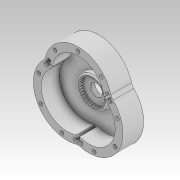
# Autodesk Inventor part: Housing
Saved by Autodesk Inventor 2020 (Build 240168000, 168)
## iProperties
Created: 2022-01-08
Part Number: Housing
Material: Generic
Document SubType Name: Modeling
Designer: DDeGo
Density: 1 g/cm^3
Appearance: Default
Author: DDeGo
Autodesk Inventor part; units mm, degrees
(part 1 of 2)
ref_plane "YZ Plane" through (0, 0, 0) normal (1, 0, 0) x (0, 1, 0)
ref_plane "XZ Plane" through (0, 0, 0) normal (0, 1, 0) x (-1, 0, 0)
ref_plane "XY Plane" through (0, 0, 0) normal (0, 0, 1) x (1, 0, 0)
sketch "Block1" plane through (0, 0, 0) normal (0, 0, 1) x (1, 0, 0)
  arc A0 (4.8525, -6.0461) -> (5.1116, -5.8287) centre (0, 0) ccw
  arc A1 (4.1606, -5.6743) -> (4.8525, -6.0461) centre (5.9978, -3.0847) ccw
  arc A2 (3.9091, -5.8504) -> (4.1606, -5.6743) centre (0, 0) ccw
  arc A3 (4.0218, -6.6277) -> (3.9091, -5.8504) centre (0.8473, -6.6911) ccw
  arc A4 (3.7289, -6.7968) -> (4.0218, -6.6277) centre (0, 0) ccw
  arc A5 (3.112, -6.3106) -> (3.7289, -6.7968) centre (5.371, -4.0793) ccw
  arc A6 (2.8338, -6.4403) -> (3.112, -6.3106) centre (0, 0) ccw
  arc A7 (2.8098, -7.2254) -> (2.8338, -6.4403) centre (-0.3275, -6.7366) ccw
  arc A8 (2.492, -7.3411) -> (2.8098, -7.2254) centre (0, 0) ccw
  arc A9 (2.8367, -7.2471) -> (2.8656, -6.4591) centre (-0.3275, -6.7366) ccw
  arc A10 (2.8656, -6.4591) -> (3.1059, -6.347) centre (0, 0) ccw
  arc A11 (3.1059, -6.347) -> (3.7282, -6.8314) centre (5.371, -4.0793) ccw
  arc A12 (3.7282, -6.8314) -> (4.0521, -6.6444) centre (0, 0) ccw
  arc A13 (4.0521, -6.6444) -> (3.9437, -5.8633) centre (0.8473, -6.6911) ccw
  arc A14 (3.9437, -5.8633) -> (4.1609, -5.7112) centre (0, 0) ccw
  arc A15 (4.1609, -5.7112) -> (4.8578, -6.0802) centre (5.9978, -3.0847) ccw
  arc A16 (4.8578, -6.0802) -> (5.1443, -5.8398) centre (0, 0) ccw
  arc A17 (2.4853, -7.375) -> (2.8367, -7.2471) centre (0, 0) ccw
  arc A18 (6.0461, -4.8525) -> (5.6743, -4.1606) centre (3.0847, -5.9978) ccw
  arc A19 (6.0802, -4.8578) -> (5.7112, -4.1609) centre (3.0847, -5.9978) ccw
  arc A20 (5.8287, -5.1116) -> (6.0461, -4.8525) centre (0, 0) ccw
  arc A21 (5.8398, -5.1443) -> (6.0802, -4.8578) centre (0, 0) ccw
  arc A22 (5.0827, -4.8656) -> (5.8287, -5.1116) centre (6.4423, -1.9963) ccw
  arc A23 (5.0894, -4.9019) -> (5.8398, -5.1443) centre (6.4423, -1.9963) ccw
  arc A24 (4.9019, -5.0894) -> (5.0894, -4.9019) centre (0, 0) ccw
  arc A25 (4.8656, -5.0827) -> (5.0827, -4.8656) centre (0, 0) ccw
  arc A26 (5.1443, -5.8398) -> (4.9019, -5.0894) centre (1.9963, -6.4423) ccw
  arc A27 (5.1116, -5.8287) -> (4.8656, -5.0827) centre (1.9963, -6.4423) ccw
  arc A28 (1.9689, -6.7551) -> (2.492, -7.3411) centre (4.5811, -4.95) ccw
  arc A29 (1.6724, -6.8346) -> (1.9689, -6.7551) centre (0, 0) ccw
  arc A30 (1.5124, -7.6036) -> (1.6724, -6.8346) centre (-1.4923, -6.5774) ccw
  arc A31 (1.1793, -7.6623) -> (1.5124, -7.6036) centre (0, 0) ccw
  arc A32 (0.7478, -7.0265) -> (1.1669, -7.6945) centre (3.6519, -5.6703) ccw
  arc A33 (0.766, -6.9944) -> (1.1793, -7.6623) centre (3.6519, -5.6703) ccw
  arc A34 (1.1669, -7.6945) -> (1.5352, -7.6296) centre (0, 0) ccw
  arc A35 (1.5352, -7.6296) -> (1.7005, -6.8585) centre (-1.4923, -6.5774) ccw
  arc A36 (1.7005, -6.8585) -> (1.9566, -6.7899) centre (0, 0) ccw
  arc A37 (1.9566, -6.7899) -> (2.4853, -7.375) centre (4.5811, -4.95) ccw
  arc A38 (5.7112, -4.1609) -> (5.8633, -3.9437) centre (0, 0) ccw
  arc A39 (5.6743, -4.1606) -> (5.8504, -3.9091) centre (0, 0) ccw
  arc A40 (5.8633, -3.9437) -> (6.6444, -4.0521) centre (6.6911, -0.8473) ccw
  arc A41 (5.8504, -3.9091) -> (6.6277, -4.0218) centre (6.6911, -0.8473) ccw
  arc A42 (6.6444, -4.0521) -> (6.8314, -3.7282) centre (0, 0) ccw
  arc A43 (6.7968, -3.7289) -> (6.3106, -3.112) centre (4.0793, -5.371) ccw
  arc A44 (6.8314, -3.7282) -> (6.347, -3.1059) centre (4.0793, -5.371) ccw
  arc A45 (6.6277, -4.0218) -> (6.7968, -3.7289) centre (0, 0) ccw
  arc A46 (-0.1691, -7.7507) -> (0.1691, -7.7507) centre (0, 0) ccw
  arc A47 (-0.4602, -7.0211) -> (-0.1691, -7.7507) centre (2.6118, -6.2183) ccw
  arc A48 (-1.7005, -6.8585) -> (-1.5352, -7.6296) centre (1.4923, -6.5774) ccw
  arc A49 (-1.6724, -6.8346) -> (-1.5124, -7.6036) centre (1.4923, -6.5774) ccw
  arc A50 (-1.5124, -7.6036) -> (-1.1793, -7.6623) centre (0, 0) ccw
  arc A51 (-1.1793, -7.6623) -> (-0.766, -6.9944) centre (-3.6519, -5.6703) ccw
  arc A52 (-1.1669, -7.6945) -> (-0.7478, -7.0265) centre (-3.6519, -5.6703) ccw
  arc A53 (-0.7478, -7.0265) -> (-0.4837, -7.0496) centre (0, 0) ccw
  arc A54 (-0.766, -6.9944) -> (-0.4602, -7.0211) centre (0, 0) ccw
  arc A55 (-0.4837, -7.0496) -> (-0.187, -7.7803) centre (2.6118, -6.2183) ccw
  arc A56 (0.4602, -7.0211) -> (0.766, -6.9944) centre (0, 0) ccw
  arc A57 (0.4837, -7.0496) -> (0.7478, -7.0265) centre (0, 0) ccw
  arc A58 (0.1691, -7.7507) -> (0.4602, -7.0211) centre (-2.6118, -6.2183) ccw
  arc A59 (0.187, -7.7803) -> (0.4837, -7.0496) centre (-2.6118, -6.2183) ccw
  arc A60 (-0.187, -7.7803) -> (0.187, -7.7803) centre (0, 0) ccw
  arc A61 (-1.5352, -7.6296) -> (-1.1669, -7.6945) centre (0, 0) ccw
  arc A62 (-1.9566, -6.7899) -> (-1.7005, -6.8585) centre (0, 0) ccw
  arc A63 (-1.9689, -6.7551) -> (-1.6724, -6.8346) centre (0, 0) ccw
  arc A64 (-2.4853, -7.375) -> (-1.9566, -6.7899) centre (-4.5811, -4.95) ccw
  arc A65 (-2.492, -7.3411) -> (-1.9689, -6.7551) centre (-4.5811, -4.95) ccw
  arc A66 (6.9944, -0.766) -> (7.0211, -0.4602) centre (0, 0) ccw
  arc A67 (7.6623, -1.1793) -> (6.9944, -0.766) centre (5.6703, -3.6519) ccw
  arc A68 (7.6036, -1.5124) -> (7.6623, -1.1793) centre (0, 0) ccw
  arc A69 (6.8346, -1.6724) -> (7.6036, -1.5124) centre (6.5774, 1.4923) ccw
  arc A70 (6.7551, -1.9689) -> (6.8346, -1.6724) centre (0, 0) ccw
  arc A71 (7.3411, -2.492) -> (6.7551, -1.9689) centre (4.95, -4.5811) ccw
  arc A72 (7.2254, -2.8098) -> (7.3411, -2.492) centre (0, 0) ccw
  arc A73 (6.4403, -2.8338) -> (7.2254, -2.8098) centre (6.7366, 0.3275) ccw
  arc A74 (6.3106, -3.112) -> (6.4403, -2.8338) centre (0, 0) ccw
  arc A75 (6.4591, -2.8656) -> (7.2471, -2.8367) centre (6.7366, 0.3275) ccw
  arc A76 (7.2471, -2.8367) -> (7.375, -2.4853) centre (0, 0) ccw
  arc A77 (6.7899, -1.9566) -> (6.8585, -1.7005) centre (0, 0) ccw
  arc A78 (7.375, -2.4853) -> (6.7899, -1.9566) centre (4.95, -4.5811) ccw
  arc A79 (6.8585, -1.7005) -> (7.6296, -1.5352) centre (6.5774, 1.4923) ccw
  arc A80 (7.6296, -1.5352) -> (7.6945, -1.1669) centre (0, 0) ccw
  arc A81 (7.6945, -1.1669) -> (7.0265, -0.7478) centre (5.6703, -3.6519) ccw
  arc A82 (7.0265, -0.7478) -> (7.0496, -0.4837) centre (0, 0) ccw
  arc A83 (6.347, -3.1059) -> (6.4591, -2.8656) centre (0, 0) ccw
  arc A84 (-3.9091, -5.8504) -> (-4.0218, -6.6277) centre (-0.8473, -6.6911) ccw
  arc A85 (-4.0218, -6.6277) -> (-3.7289, -6.7968) centre (0, 0) ccw
  arc A86 (-4.0521, -6.6444) -> (-3.7282, -6.8314) centre (0, 0) ccw
  arc A87 (-3.1059, -6.347) -> (-2.8656, -6.4591) centre (0, 0) ccw
  arc A88 (-3.7289, -6.7968) -> (-3.112, -6.3106) centre (-5.371, -4.0793) ccw
  arc A89 (-3.112, -6.3106) -> (-2.8338, -6.4403) centre (0, 0) ccw
  arc A90 (-3.7282, -6.8314) -> (-3.1059, -6.347) centre (-5.371, -4.0793) ccw
  arc A91 (-2.8338, -6.4403) -> (-2.8098, -7.2254) centre (0.3275, -6.7366) ccw
  arc A92 (-2.8656, -6.4591) -> (-2.8367, -7.2471) centre (0.3275, -6.7366) ccw
  arc A93 (-2.8098, -7.2254) -> (-2.492, -7.3411) centre (0, 0) ccw
  arc A94 (-2.8367, -7.2471) -> (-2.4853, -7.375) centre (0, 0) ccw
  arc A95 (-3.9437, -5.8633) -> (-4.0521, -6.6444) centre (-0.8473, -6.6911) ccw
  arc A96 (-4.1609, -5.7112) -> (-3.9437, -5.8633) centre (0, 0) ccw
  arc A97 (-4.8578, -6.0802) -> (-4.1609, -5.7112) centre (-5.9978, -3.0847) ccw
  arc A98 (-4.8525, -6.0461) -> (-4.1606, -5.6743) centre (-5.9978, -3.0847) ccw
  arc A99 (-5.1116, -5.8287) -> (-4.8525, -6.0461) centre (0, 0) ccw
  arc A100 (-5.1443, -5.8398) -> (-4.8578, -6.0802) centre (0, 0) ccw
  arc A101 (-4.8656, -5.0827) -> (-5.1116, -5.8287) centre (-1.9963, -6.4423) ccw
  arc A102 (-4.9019, -5.0894) -> (-5.1443, -5.8398) centre (-1.9963, -6.4423) ccw
  arc A103 (-4.1606, -5.6743) -> (-3.9091, -5.8504) centre (0, 0) ccw
  arc A104 (6.8346, 1.6724) -> (6.7551, 1.9689) centre (0, 0) ccw
  arc A105 (7.6036, 1.5124) -> (6.8346, 1.6724) centre (6.5774, -1.4923) ccw
  arc A106 (7.6623, 1.1793) -> (7.6036, 1.5124) centre (0, 0) ccw
  arc A107 (6.9944, 0.766) -> (7.6623, 1.1793) centre (5.6703, 3.6519) ccw
  arc A108 (7.0211, 0.4602) -> (6.9944, 0.766) centre (0, 0) ccw
  arc A109 (7.7507, 0.1691) -> (7.0211, 0.4602) centre (6.2183, -2.6118) ccw
  arc A110 (7.7507, -0.1691) -> (7.7507, 0.1691) centre (0, 0) ccw
  arc A111 (7.0211, -0.4602) -> (7.7507, -0.1691) centre (6.2183, 2.6118) ccw
  arc A112 (6.8585, 1.7005) -> (6.7899, 1.9566) centre (0, 0) ccw
  arc A113 (7.0496, 0.4837) -> (7.0265, 0.7478) centre (0, 0) ccw
  arc A114 (7.6296, 1.5352) -> (6.8585, 1.7005) centre (6.5774, -1.4923) ccw
  arc A115 (7.6945, 1.1669) -> (7.6296, 1.5352) centre (0, 0) ccw
  arc A116 (7.0265, 0.7478) -> (7.6945, 1.1669) centre (5.6703, 3.6519) ccw
  arc A117 (7.7803, 0.187) -> (7.0496, 0.4837) centre (6.2183, -2.6118) ccw
  arc A118 (7.0496, -0.4837) -> (7.7803, -0.187) centre (6.2183, 2.6118) ccw
  arc A119 (7.7803, -0.187) -> (7.7803, 0.187) centre (0, 0) ccw
  arc A120 (-5.0827, -4.8656) -> (-4.8656, -5.0827) centre (0, 0) ccw
  arc A121 (-5.8287, -5.1116) -> (-5.0827, -4.8656) centre (-6.4423, -1.9963) ccw
  arc A122 (-6.0461, -4.8525) -> (-5.8287, -5.1116) centre (0, 0) ccw
  arc A123 (-5.6743, -4.1606) -> (-6.0461, -4.8525) centre (-3.0847, -5.9978) ccw
  arc A124 (-5.8504, -3.9091) -> (-5.6743, -4.1606) centre (0, 0) ccw
  arc A125 (-6.6277, -4.0218) -> (-5.8504, -3.9091) centre (-6.6911, -0.8473) ccw
  arc A126 (-6.7968, -3.7289) -> (-6.6277, -4.0218) centre (0, 0) ccw
  arc A127 (-6.3106, -3.112) -> (-6.7968, -3.7289) centre (-4.0793, -5.371) ccw
  arc A128 (-6.4403, -2.8338) -> (-6.3106, -3.112) centre (0, 0) ccw
  arc A129 (-6.4591, -2.8656) -> (-6.347, -3.1059) centre (0, 0) ccw
  arc A130 (-6.347, -3.1059) -> (-6.8314, -3.7282) centre (-4.0793, -5.371) ccw
  arc A131 (-6.8314, -3.7282) -> (-6.6444, -4.0521) centre (0, 0) ccw
  arc A132 (-6.6444, -4.0521) -> (-5.8633, -3.9437) centre (-6.6911, -0.8473) ccw
  arc A133 (-5.8633, -3.9437) -> (-5.7112, -4.1609) centre (0, 0) ccw
  arc A134 (-5.7112, -4.1609) -> (-6.0802, -4.8578) centre (-3.0847, -5.9978) ccw
  arc A135 (-6.0802, -4.8578) -> (-5.8398, -5.1443) centre (0, 0) ccw
  arc A136 (-5.0894, -4.9019) -> (-4.9019, -5.0894) centre (0, 0) ccw
  arc A137 (-5.8398, -5.1443) -> (-5.0894, -4.9019) centre (-6.4423, -1.9963) ccw
  arc A138 (5.6743, 4.1606) -> (6.0461, 4.8525) centre (3.0847, 5.9978) ccw
  arc A139 (5.8504, 3.9091) -> (5.6743, 4.1606) centre (0, 0) ccw
  arc A140 (6.6277, 4.0218) -> (5.8504, 3.9091) centre (6.6911, 0.8473) ccw
  arc A141 (6.7968, 3.7289) -> (6.6277, 4.0218) centre (0, 0) ccw
  arc A142 (6.3106, 3.112) -> (6.7968, 3.7289) centre (4.0793, 5.371) ccw
  arc A143 (6.4403, 2.8338) -> (6.3106, 3.112) centre (0, 0) ccw
  arc A144 (7.2254, 2.8098) -> (6.4403, 2.8338) centre (6.7366, -0.3275) ccw
  arc A145 (7.3411, 2.492) -> (7.2254, 2.8098) centre (0, 0) ccw
  arc A146 (6.7551, 1.9689) -> (7.3411, 2.492) centre (4.95, 4.5811) ccw
  arc A147 (6.7899, 1.9566) -> (7.375, 2.4853) centre (4.95, 4.5811) ccw
  arc A148 (7.375, 2.4853) -> (7.2471, 2.8367) centre (0, 0) ccw
  arc A149 (7.2471, 2.8367) -> (6.4591, 2.8656) centre (6.7366, -0.3275) ccw
  arc A150 (6.4591, 2.8656) -> (6.347, 3.1059) centre (0, 0) ccw
  arc A151 (6.8314, 3.7282) -> (6.6444, 4.0521) centre (0, 0) ccw
  arc A152 (6.6444, 4.0521) -> (5.8633, 3.9437) centre (6.6911, 0.8473) ccw
  arc A153 (5.8633, 3.9437) -> (5.7112, 4.1609) centre (0, 0) ccw
  arc A154 (5.7112, 4.1609) -> (6.0802, 4.8578) centre (3.0847, 5.9978) ccw
  arc A155 (6.347, 3.1059) -> (6.8314, 3.7282) centre (4.0793, 5.371) ccw
  arc A156 (-7.2254, -2.8098) -> (-6.4403, -2.8338) centre (-6.7366, 0.3275) ccw
  arc A157 (-7.3411, -2.492) -> (-7.2254, -2.8098) centre (0, 0) ccw
  arc A158 (-6.7551, -1.9689) -> (-7.3411, -2.492) centre (-4.95, -4.5811) ccw
  arc A159 (-6.8346, -1.6724) -> (-6.7551, -1.9689) centre (0, 0) ccw
  arc A160 (-7.6036, -1.5124) -> (-6.8346, -1.6724) centre (-6.5774, 1.4923) ccw
  arc A161 (-7.6623, -1.1793) -> (-7.6036, -1.5124) centre (0, 0) ccw
  arc A162 (-6.9944, -0.766) -> (-7.6623, -1.1793) centre (-5.6703, -3.6519) ccw
  arc A163 (-7.0211, -0.4602) -> (-6.9944, -0.766) centre (0, 0) ccw
  arc A164 (-7.0496, -0.4837) -> (-7.0265, -0.7478) centre (0, 0) ccw
  arc A165 (-7.0265, -0.7478) -> (-7.6945, -1.1669) centre (-5.6703, -3.6519) ccw
  arc A166 (-7.6945, -1.1669) -> (-7.6296, -1.5352) centre (0, 0) ccw
  arc A167 (-7.6296, -1.5352) -> (-6.8585, -1.7005) centre (-6.5774, 1.4923) ccw
  arc A168 (-6.8585, -1.7005) -> (-6.7899, -1.9566) centre (0, 0) ccw
  arc A169 (-6.7899, -1.9566) -> (-7.375, -2.4853) centre (-4.95, -4.5811) ccw
  arc A170 (-7.2471, -2.8367) -> (-6.4591, -2.8656) centre (-6.7366, 0.3275) ccw
  arc A171 (-7.375, -2.4853) -> (-7.2471, -2.8367) centre (0, 0) ccw
  arc A172 (4.0218, 6.6277) -> (3.7289, 6.7968) centre (0, 0) ccw
  arc A173 (3.9091, 5.8504) -> (4.0218, 6.6277) centre (0.8473, 6.6911) ccw
  arc A174 (4.1606, 5.6743) -> (3.9091, 5.8504) centre (0, 0) ccw
  arc A175 (4.8525, 6.0461) -> (4.1606, 5.6743) centre (5.9978, 3.0847) ccw
  arc A176 (5.1116, 5.8287) -> (4.8525, 6.0461) centre (0, 0) ccw
  arc A177 (4.8656, 5.0827) -> (5.1116, 5.8287) centre (1.9963, 6.4423) ccw
  arc A178 (5.0827, 4.8656) -> (4.8656, 5.0827) centre (0, 0) ccw
  arc A179 (5.8287, 5.1116) -> (5.0827, 4.8656) centre (6.4423, 1.9963) ccw
  arc A180 (6.0461, 4.8525) -> (5.8287, 5.1116) centre (0, 0) ccw
  arc A181 (6.0802, 4.8578) -> (5.8398, 5.1443) centre (0, 0) ccw
  arc A182 (5.8398, 5.1443) -> (5.0894, 4.9019) centre (6.4423, 1.9963) ccw
  arc A183 (5.0894, 4.9019) -> (4.9019, 5.0894) centre (0, 0) ccw
  arc A184 (4.9019, 5.0894) -> (5.1443, 5.8398) centre (1.9963, 6.4423) ccw
  arc A185 (5.1443, 5.8398) -> (4.8578, 6.0802) centre (0, 0) ccw
  arc A186 (4.1609, 5.7112) -> (3.9437, 5.8633) centre (0, 0) ccw
  arc A187 (4.8578, 6.0802) -> (4.1609, 5.7112) centre (5.9978, 3.0847) ccw
  arc A188 (3.9437, 5.8633) -> (4.0521, 6.6444) centre (0.8473, 6.6911) ccw
  arc A189 (4.0521, 6.6444) -> (3.7282, 6.8314) centre (0, 0) ccw
  arc A190 (1.5124, 7.6036) -> (1.1793, 7.6623) centre (0, 0) ccw
  arc A191 (1.6724, 6.8346) -> (1.5124, 7.6036) centre (-1.4923, 6.5774) ccw
  arc A192 (1.9689, 6.7551) -> (1.6724, 6.8346) centre (0, 0) ccw
  arc A193 (2.492, 7.3411) -> (1.9689, 6.7551) centre (4.5811, 4.95) ccw
  arc A194 (2.8098, 7.2254) -> (2.492, 7.3411) centre (0, 0) ccw
  arc A195 (2.8338, 6.4403) -> (2.8098, 7.2254) centre (-0.3275, 6.7366) ccw
  arc A196 (3.112, 6.3106) -> (2.8338, 6.4403) centre (0, 0) ccw
  arc A197 (3.7289, 6.7968) -> (3.112, 6.3106) centre (5.371, 4.0793) ccw
  arc A198 (3.7282, 6.8314) -> (3.1059, 6.347) centre (5.371, 4.0793) ccw
  arc A199 (3.1059, 6.347) -> (2.8656, 6.4591) centre (0, 0) ccw
  arc A200 (2.8367, 7.2471) -> (2.4853, 7.375) centre (0, 0) ccw
  arc A201 (1.9566, 6.7899) -> (1.7005, 6.8585) centre (0, 0) ccw
  arc A202 (2.4853, 7.375) -> (1.9566, 6.7899) centre (4.5811, 4.95) ccw
  arc A203 (1.7005, 6.8585) -> (1.5352, 7.6296) centre (-1.4923, 6.5774) ccw
  arc A204 (1.5352, 7.6296) -> (1.1669, 7.6945) centre (0, 0) ccw
  arc A205 (2.8656, 6.4591) -> (2.8367, 7.2471) centre (-0.3275, 6.7366) ccw
  circle A206 centre (0, 0) radius 8.5 construction
  arc A207 (-1.5124, 7.6036) -> (-1.6724, 6.8346) centre (1.4923, 6.5774) ccw
  arc A208 (-1.1793, 7.6623) -> (-1.5124, 7.6036) centre (0, 0) ccw
  arc A209 (-0.766, 6.9944) -> (-1.1793, 7.6623) centre (-3.6519, 5.6703) ccw
  arc A210 (-0.4602, 7.0211) -> (-0.766, 6.9944) centre (0, 0) ccw
  arc A211 (-0.1691, 7.7507) -> (-0.4602, 7.0211) centre (2.6118, 6.2183) ccw
  arc A212 (0.1691, 7.7507) -> (-0.1691, 7.7507) centre (0, 0) ccw
  arc A213 (0.4602, 7.0211) -> (0.1691, 7.7507) centre (-2.6118, 6.2183) ccw
  arc A214 (0.766, 6.9944) -> (0.4602, 7.0211) centre (0, 0) ccw
  arc A215 (1.1793, 7.6623) -> (0.766, 6.9944) centre (3.6519, 5.6703) ccw
  arc A216 (1.1669, 7.6945) -> (0.7478, 7.0265) centre (3.6519, 5.6703) ccw
  arc A217 (0.7478, 7.0265) -> (0.4837, 7.0496) centre (0, 0) ccw
  arc A218 (0.4837, 7.0496) -> (0.187, 7.7803) centre (-2.6118, 6.2183) ccw
  arc A219 (0.187, 7.7803) -> (-0.187, 7.7803) centre (0, 0) ccw
  arc A220 (-0.187, 7.7803) -> (-0.4837, 7.0496) centre (2.6118, 6.2183) ccw
  arc A221 (-0.4837, 7.0496) -> (-0.7478, 7.0265) centre (0, 0) ccw
  arc A222 (-0.7478, 7.0265) -> (-1.1669, 7.6945) centre (-3.6519, 5.6703) ccw
  arc A223 (-1.1669, 7.6945) -> (-1.5352, 7.6296) centre (0, 0) ccw
  arc A224 (-1.5352, 7.6296) -> (-1.7005, 6.8585) centre (1.4923, 6.5774) ccw
  arc A225 (-7.7507, -0.1691) -> (-7.0211, -0.4602) centre (-6.2183, 2.6118) ccw
  arc A226 (-7.7507, 0.1691) -> (-7.7507, -0.1691) centre (0, 0) ccw
  arc A227 (-7.0211, 0.4602) -> (-7.7507, 0.1691) centre (-6.2183, -2.6118) ccw
  arc A228 (-6.9944, 0.766) -> (-7.0211, 0.4602) centre (0, 0) ccw
  arc A229 (-7.6623, 1.1793) -> (-6.9944, 0.766) centre (-5.6703, 3.6519) ccw
  arc A230 (-7.6036, 1.5124) -> (-7.6623, 1.1793) centre (0, 0) ccw
  arc A231 (-6.8346, 1.6724) -> (-7.6036, 1.5124) centre (-6.5774, -1.4923) ccw
  arc A232 (-6.7551, 1.9689) -> (-6.8346, 1.6724) centre (0, 0) ccw
  arc A233 (-6.7899, 1.9566) -> (-6.8585, 1.7005) centre (0, 0) ccw
  arc A234 (-6.8585, 1.7005) -> (-7.6296, 1.5352) centre (-6.5774, -1.4923) ccw
  arc A235 (-7.6296, 1.5352) -> (-7.6945, 1.1669) centre (0, 0) ccw
  arc A236 (-7.6945, 1.1669) -> (-7.0265, 0.7478) centre (-5.6703, 3.6519) ccw
  arc A237 (-7.0265, 0.7478) -> (-7.0496, 0.4837) centre (0, 0) ccw
  arc A238 (-7.0496, 0.4837) -> (-7.7803, 0.187) centre (-6.2183, -2.6118) ccw
  arc A239 (-7.7803, 0.187) -> (-7.7803, -0.187) centre (0, 0) ccw
  arc A240 (-7.7803, -0.187) -> (-7.0496, -0.4837) centre (-6.2183, 2.6118) ccw
  arc A241 (-4.0218, 6.6277) -> (-3.9091, 5.8504) centre (-0.8473, 6.6911) ccw
  arc A242 (-3.7289, 6.7968) -> (-4.0218, 6.6277) centre (0, 0) ccw
  arc A243 (-3.112, 6.3106) -> (-3.7289, 6.7968) centre (-5.371, 4.0793) ccw
  arc A244 (-2.8338, 6.4403) -> (-3.112, 6.3106) centre (0, 0) ccw
  arc A245 (-2.8098, 7.2254) -> (-2.8338, 6.4403) centre (0.3275, 6.7366) ccw
  arc A246 (-2.492, 7.3411) -> (-2.8098, 7.2254) centre (0, 0) ccw
  arc A247 (-1.9689, 6.7551) -> (-2.492, 7.3411) centre (-4.5811, 4.95) ccw
  arc A248 (-1.6724, 6.8346) -> (-1.9689, 6.7551) centre (0, 0) ccw
  arc A249 (-1.7005, 6.8585) -> (-1.9566, 6.7899) centre (0, 0) ccw
  arc A250 (-1.9566, 6.7899) -> (-2.4853, 7.375) centre (-4.5811, 4.95) ccw
  arc A251 (-2.4853, 7.375) -> (-2.8367, 7.2471) centre (0, 0) ccw
  arc A252 (-2.8367, 7.2471) -> (-2.8656, 6.4591) centre (0.3275, 6.7366) ccw
  arc A253 (-2.8656, 6.4591) -> (-3.1059, 6.347) centre (0, 0) ccw
  arc A254 (-3.1059, 6.347) -> (-3.7282, 6.8314) centre (-5.371, 4.0793) ccw
  arc A255 (-3.7282, 6.8314) -> (-4.0521, 6.6444) centre (0, 0) ccw
  arc A256 (-4.0521, 6.6444) -> (-3.9437, 5.8633) centre (-0.8473, 6.6911) ccw
  arc A257 (-6.0461, 4.8525) -> (-5.6743, 4.1606) centre (-3.0847, 5.9978) ccw
  arc A258 (-5.8287, 5.1116) -> (-6.0461, 4.8525) centre (0, 0) ccw
  arc A259 (-5.0827, 4.8656) -> (-5.8287, 5.1116) centre (-6.4423, 1.9963) ccw
  arc A260 (-4.8656, 5.0827) -> (-5.0827, 4.8656) centre (0, 0) ccw
  arc A261 (-5.1116, 5.8287) -> (-4.8656, 5.0827) centre (-1.9963, 6.4423) ccw
  arc A262 (-4.8525, 6.0461) -> (-5.1116, 5.8287) centre (0, 0) ccw
  arc A263 (-4.1606, 5.6743) -> (-4.8525, 6.0461) centre (-5.9978, 3.0847) ccw
  arc A264 (-3.9091, 5.8504) -> (-4.1606, 5.6743) centre (0, 0) ccw
  arc A265 (-3.9437, 5.8633) -> (-4.1609, 5.7112) centre (0, 0) ccw
  arc A266 (-4.1609, 5.7112) -> (-4.8578, 6.0802) centre (-5.9978, 3.0847) ccw
  arc A267 (-4.8578, 6.0802) -> (-5.1443, 5.8398) centre (0, 0) ccw
  arc A268 (-4.9019, 5.0894) -> (-5.0894, 4.9019) centre (0, 0) ccw
  arc A269 (-5.0894, 4.9019) -> (-5.8398, 5.1443) centre (-6.4423, 1.9963) ccw
  arc A270 (-5.8398, 5.1443) -> (-6.0802, 4.8578) centre (0, 0) ccw
  arc A271 (-6.0802, 4.8578) -> (-5.7112, 4.1609) centre (-3.0847, 5.9978) ccw
  arc A272 (-5.1443, 5.8398) -> (-4.9019, 5.0894) centre (-1.9963, 6.4423) ccw
  arc A273 (-7.3411, 2.492) -> (-6.7551, 1.9689) centre (-4.95, 4.5811) ccw
  arc A274 (-7.2254, 2.8098) -> (-7.3411, 2.492) centre (0, 0) ccw
  arc A275 (-6.4403, 2.8338) -> (-7.2254, 2.8098) centre (-6.7366, -0.3275) ccw
  arc A276 (-6.3106, 3.112) -> (-6.4403, 2.8338) centre (0, 0) ccw
  arc A277 (-6.7968, 3.7289) -> (-6.3106, 3.112) centre (-4.0793, 5.371) ccw
  arc A278 (-6.6277, 4.0218) -> (-6.7968, 3.7289) centre (0, 0) ccw
  arc A279 (-5.8504, 3.9091) -> (-6.6277, 4.0218) centre (-6.6911, 0.8473) ccw
  arc A280 (-5.6743, 4.1606) -> (-5.8504, 3.9091) centre (0, 0) ccw
  arc A281 (-5.7112, 4.1609) -> (-5.8633, 3.9437) centre (0, 0) ccw
  arc A282 (-5.8633, 3.9437) -> (-6.6444, 4.0521) centre (-6.6911, 0.8473) ccw
  arc A283 (-6.6444, 4.0521) -> (-6.8314, 3.7282) centre (0, 0) ccw
  arc A284 (-6.8314, 3.7282) -> (-6.347, 3.1059) centre (-4.0793, 5.371) ccw
  arc A285 (-6.347, 3.1059) -> (-6.4591, 2.8656) centre (0, 0) ccw
  arc A286 (-6.4591, 2.8656) -> (-7.2471, 2.8367) centre (-6.7366, -0.3275) ccw
  arc A287 (-7.2471, 2.8367) -> (-7.375, 2.4853) centre (0, 0) ccw
  arc A288 (-7.375, 2.4853) -> (-6.7899, 1.9566) centre (-4.95, 4.5811) ccw
  point P0 (0, 0)
  dimension "d15" = 0.03
  measures "d15" radial gap between concentric circles of A91 A92
derived "LP2_master.ipt"
sketch "ChamberWalls" plane through (0, 0, 0) normal (0, 0, 1) x (1, 0, 0)
  arc A0 (-8.6566, -4.9979) -> (14.9371, 8.624) centre (0, 7.2521) ccw construction
  arc A1 (0, -17.2479) -> (14.9371, 8.624) centre (6.2805, -3.626) ccw
  arc A2 (-14.9371, 8.624) -> (0, -17.2479) centre (-6.2805, -3.626) ccw
  line L0 (-6.2805, -3.626) -> (0, 0) construction
  line L1 (0, 0) -> (0, 7.2521) construction
  line L2 (0, 0) -> (6.2805, -3.626) construction
  arc A3 (0, 9.9958) -> (-14.9371, 8.624) centre (-6.2805, -3.626) ccw construction
  arc A4 (-14.9371, 8.624) -> (-8.6566, -4.9979) centre (0, 7.2521) ccw construction
  arc A5 (-8.6566, -4.9979) -> (0, -17.2479) centre (6.2805, -3.626) ccw construction
  arc A6 (0, -17.2479) -> (0, 9.9958) centre (-6.2805, -3.626) ccw construction
  arc A7 (14.9371, 8.624) -> (-14.9371, 8.624) centre (0, 7.2521) ccw
  arc A8 (14.9371, 8.624) -> (-8.6566, -4.9979) centre (6.2805, -3.626) ccw construction
  point P0 (19.2709, -11.126)
sketch "HousingWalls" plane through (0, 0, -1.5) normal (0, 0, 1) x (1, 0, 0)
  arc A0 (14.9371, 8.624) -> (-14.9371, 8.624) centre (0, 7.2521) ccw construction
  arc A1 (-14.9371, 8.624) -> (0, -17.2479) centre (-6.2805, -3.626) ccw construction
  arc A2 (0, -17.2479) -> (14.9371, 8.624) centre (6.2805, -3.626) ccw construction
  arc A3 (-20.1043, 10.1272) -> (-1.2817, -22.4744) centre (-6.2805, -3.626) ccw
  arc A4 (18.8226, 12.3472) -> (-18.8226, 12.3472) centre (0, 7.2521) ccw
  arc A5 (1.2817, -22.4744) -> (20.1043, 10.1272) centre (6.2805, -3.626) ccw
  arc A6 (-20.1043, 10.1272) -> (-18.8226, 12.3472) centre (-23.6489, 13.6537) ccw
  arc A7 (18.8226, 12.3472) -> (20.1043, 10.1272) centre (23.6489, 13.6537) ccw
  arc A8 (1.2817, -22.4744) -> (-1.2817, -22.4744) centre (0, -27.3074) ccw
  point P0 (0, 0)
sketch "ApexCut" plane through (0, 0, 0) normal (0, 0, 1) x (1, 0, 0)
  line L0 (0, 0) -> (-15.6733, 9.049) construction
  circle A0 centre (-15.6733, 9.049) radius 0.85 construction
  line L1 (-15.6733, 9.049) -> (-15.2483, 9.7851) construction
  line L2 (-15.2483, 9.7851) -> (-16.34, 10.4154)
  line L3 (-16.34, 10.4154) -> (-15.49, 11.8876)
  line L4 (-15.49, 11.8876) -> (-17.222, 12.8876)
  line L5 (-17.222, 12.8876) -> (-19.772, 8.4709)
  line L6 (-19.772, 8.4709) -> (-18.04, 7.4709)
  line L7 (-18.04, 7.4709) -> (-17.19, 8.9431)
  line L8 (-17.19, 8.9431) -> (-16.0983, 8.3128)
  line L9 (-17.19, 8.9431) -> (-16.34, 10.4154) construction
  line L10 (-16.0983, 8.3128) -> (-15.6733, 9.049) construction
  line L11 (-16.0983, 8.3128) -> (-15.3621, 7.8878)
  line L12 (-15.3621, 7.8878) -> (-14.5121, 9.3601)
  line L13 (-14.5121, 9.3601) -> (-15.2483, 9.7851)
  arc A1 (-14.9371, 8.624) -> (0, -17.2479) centre (-6.2805, -3.626) ccw construction
  point P0 (-15.6744, 8.0681)
ref_plane "Chamber_bot" through (0, 0, 0) normal (0, 0, 1) x (1, 0, 0)
ref_plane "Housing_bot" through (0, 0, -1.5) normal (0, 0, 1) x (1, 0, 0)
ref_plane "Rotor_bot" through (0, 0, -0.2) normal (0, 0, 1) x (1, 0, 0)
ref_plane "RotorFlat_bot" through (0, 0, 0.3) normal (0, 0, 1) x (1, 0, 0)
ref_plane "RotorTeeth_top" through (0, 0, 3) normal (0, 0, 1) x (1, 0, 0)
ref_plane "RotorTeeth_bot" through (0, 0, 0.5) normal (0, 0, 1) x (1, 0, 0)
ref_plane "RotorBearinggap" through (0, 0, 4) normal (0, 0, 1) x (1, 0, 0)
ref_plane "RotorBearing_bot" through (0, 0, 4.5) normal (0, 0, 1) x (1, 0, 0)
ref_plane "RotorBearing_top" through (0, 0, 8.5) normal (0, 0, 1) x (1, 0, 0)
ref_plane "RotorFlat_top" through (0, 0, 10.1) normal (0, 0, 1) x (1, 0, 0)
ref_plane "Chamber_top" through (0, 0, 10.4) normal (0, 0, 1) x (1, 0, 0)
ref_plane "HousingTeeth_top" through (0, 0, 2.5) normal (0, 0, 1) x (1, 0, 0)
sketch "HousingBoltPattern" plane through (0, 0, 10.4) normal (0, 0, 1) x (1, 0, 0)
  arc A0 (-20.1043, 10.1272) -> (-18.8226, 12.3472) centre (-23.6489, 13.6537) ccw construction
  arc A1 (18.8226, 12.3472) -> (-18.8226, 12.3472) centre (0, 7.2521) ccw construction
  arc A2 (-20.1043, 10.1272) -> (-1.2817, -22.4744) centre (-6.2805, -3.626) ccw construction
  arc A3 (18.8226, 12.3472) -> (20.1043, 10.1272) centre (23.6489, 13.6537) ccw construction
  arc A4 (1.2817, -22.4744) -> (20.1043, 10.1272) centre (6.2805, -3.626) ccw construction
  arc A5 (1.2817, -22.4744) -> (-1.2817, -22.4744) centre (0, -27.3074) ccw construction
  arc A6 (-14.9371, 8.624) -> (0, -17.2479) centre (-6.2805, -3.626) ccw construction
  arc A7 (14.9371, 8.624) -> (-14.9371, 8.624) centre (0, 7.2521) ccw construction
  arc A8 (0, -17.2479) -> (14.9371, 8.624) centre (6.2805, -3.626) ccw construction
  arc A9 (-17.1932, 9.9265) -> (0, -19.853) centre (-6.2805, -3.626) ccw construction
  arc A10 (0, -19.853) -> (17.1932, 9.9265) centre (6.2805, -3.626) ccw construction
  arc A11 (17.1932, 9.9265) -> (-17.1932, 9.9265) centre (0, 7.2521) ccw construction
  circle A12 centre (-22.6311, 2.3251) radius 1.05
  circle A13 centre (-21.3493, -12.326) radius 1.05
  circle A14 centre (-9.302, -20.7617) radius 1.05
  line L0 (-9.302, -20.7617) -> (-6.2805, -3.626) construction
  line L1 (-6.2805, -3.626) -> (-22.6311, 2.3251) construction
  line L2 (-6.2805, -3.626) -> (-21.3493, -12.326) construction
  line L3 (-6.2805, -3.626) -> (0, 0) construction
  circle A15 centre (9.302, -20.7617) radius 1.05
  circle A16 centre (21.3493, -12.326) radius 1.05
  circle A17 centre (22.6311, 2.3251) radius 1.05
  circle A18 centre (13.3292, 18.4366) radius 1.05
  circle A19 centre (0, 24.6521) radius 1.05
  circle A20 centre (-13.3292, 18.4366) radius 1.05
sketch "HousingBearing" plane through (0, 0, 0) normal (1, 0, 0) x (0, 1, 0)
  line L0 (0, 0) -> (0, -3.2)
  line L1 (0, -3.2) -> (4.025, -3.2)
  line L2 (4.025, -3.2) -> (4.525, -3.2)
  line L3 (4.525, -3.2) -> (6.551, -1.5)
  line L4 (6.551, -1.5) -> (6.551, 0) construction
  line L5 (6.551, 0) -> (3.525, 0) construction
  line L6 (4.025, -3.2) -> (4.025, -1.5)
  line L7 (4.025, -0.5) -> (3.525, -0.5)
  line L8 (3.525, -0.5) -> (3.525, 0)
  line L9 (-87.0508, -1.5) -> (84.6316, -1.5)
  line L10 (3.525, 0) -> (0, 0)
  line L11 (6.551, -1.5) -> (4.025, -1.5)
  line L12 (4.025, -1.5) -> (4.025, -0.5)
sketch "HousingTeeth" plane through (0, 0, 0) normal (1, 0, 0) x (0, 1, 0)
  line L0 (0, 0) -> (0, 2.5) construction
  line L1 (0, 2.5) -> (6, 2.5) construction
  line L2 (6, 2.5) -> (6, 0)
  line L3 (6, 0) -> (0, 0) construction
  line L4 (6, 2.5) -> (7.7327, 2.5)
  line L5 (8.6986, 1.7588) -> (9.1699, 0)
  line L6 (9.1699, 0) -> (6, 0)
  line L7 (-87.0508, 2.5) -> (84.6316, 2.5) construction
  arc A0 (8.6986, 1.7588) -> (7.7327, 2.5) centre (7.7327, 1.5) ccw
  point P0 (8.5, 2.5)
extrude "Extrusion1" add sketch "HousingWalls" along normal up to surface (1.5 mm away)
sketch "Sketch8" plane through (0, 7.2521, 0) normal (0, 0, 1) x (1, 0, 0)
  arc A0 (-14.9371, 1.3719) -> (0, -24.5) centre (-6.2805, -10.8781) ccw projected
  arc A1 (14.9371, 1.3719) -> (-14.9371, 1.3719) centre (0, 0) ccw projected
  arc A2 (0, -24.5) -> (14.9371, 1.3719) centre (6.2805, -10.8781) ccw projected
  arc A3 (-20.1043, 2.8751) -> (-1.2817, -29.7265) centre (-6.2805, -10.8781) ccw projected
  arc A4 (1.2817, -29.7265) -> (-1.2817, -29.7265) centre (0, -34.5595) ccw projected
  arc A5 (1.2817, -29.7265) -> (20.1043, 2.8751) centre (6.2805, -10.8781) ccw projected
  arc A6 (18.8226, 5.0952) -> (20.1043, 2.8751) centre (23.6489, 6.4016) ccw projected
  arc A7 (18.8226, 5.0952) -> (-18.8226, 5.0952) centre (0, 0) ccw projected
  arc A8 (-20.1043, 2.8751) -> (-18.8226, 5.0952) centre (-23.6489, 6.4016) ccw projected
  point P0 (0, -7.2521)
extrude "Extrusion2" add sketch "Sketch8" along normal up to surface (10.4 mm away)
extrude "Extrusion3" cut sketch "ApexCut" along normal through all
pattern_circular "Circular Pattern1" count 3 over 360 about axis through (0, 0, -1.5) along (0, 0, 1) of "Extrusion3"
extrude "Extrusion4" cut sketch "HousingBoltPattern" against normal through all
revolve "Revolution1" cut sketch "HousingBearing" angle 360 about axis through (0, 0, 0) along (0, 0, -1) contours L10 L8 L7 L12 L9 L0 | L9 L6 L1 L0
revolve "Revolution2" add sketch "HousingBearing" angle 360 about axis through (0, 0, 0) along (0, 0, -1) contours L9 L3 L2 L6
revolve "Revolution3" add sketch "HousingTeeth" angle 360 about axis through (0, 0, 0) along (0, 0, 1)
sketch "Sketch12" plane through (0, 0, 2.5) normal (0, 0, 1) x (1, 0, 0)
  arc A0 (5.7784, -5.1683) -> (5.9984, -4.9113) centre (0, 0) ccw
  arc A1 (5.0349, -4.915) -> (5.7784, -5.1683) centre (6.4225, -2.0591) ccw
  arc A2 (4.8157, -5.13) -> (5.0349, -4.915) centre (0, 0) ccw
  arc A3 (5.0544, -5.8783) -> (4.8157, -5.13) centre (1.9333, -6.4615) ccw
  arc A4 (4.7932, -6.0932) -> (5.0544, -5.8783) centre (0, 0) ccw
  arc A5 (4.1049, -5.7147) -> (4.7932, -6.0932) centre (5.9674, -3.1431) ccw
  arc A6 (3.8518, -5.8883) -> (4.1049, -5.7147) centre (0, 0) ccw
  arc A7 (3.9569, -6.6667) -> (3.8518, -5.8883) centre (0.7819, -6.6991) ccw
  arc A8 (3.6623, -6.8329) -> (3.9569, -6.6667) centre (0, 0) ccw
  arc A9 (3.987, -6.6837) -> (3.8862, -5.9016) centre (0.7819, -6.6991) ccw
  arc A10 (3.8862, -5.9016) -> (4.1049, -5.7516) centre (0, 0) ccw
  arc A11 (4.1049, -5.7516) -> (4.7982, -6.1274) centre (5.9674, -3.1431) ccw
  arc A12 (4.7982, -6.1274) -> (5.087, -5.8898) centre (0, 0) ccw
  arc A13 (5.087, -5.8898) -> (4.852, -5.1371) centre (1.9333, -6.4615) ccw
  arc A14 (4.852, -5.1371) -> (5.0413, -4.9514) centre (0, 0) ccw
  arc A15 (5.0413, -4.9514) -> (5.7893, -5.2011) centre (6.4225, -2.0591) ccw
  arc A16 (5.7893, -5.2011) -> (6.0325, -4.917) centre (0, 0) ccw
  arc A17 (3.6613, -6.8675) -> (3.987, -6.6837) centre (0, 0) ccw
  arc A18 (6.7601, -3.7951) -> (6.2799, -3.1735) centre (4.0266, -5.4106) ccw
  arc A19 (6.7947, -3.7947) -> (6.3164, -3.1678) centre (4.0266, -5.4106) ccw
  arc A20 (6.5881, -4.0864) -> (6.7601, -3.7951) centre (0, 0) ccw
  arc A21 (6.6045, -4.1168) -> (6.7947, -3.7947) centre (0, 0) ccw
  arc A22 (5.8119, -3.9661) -> (6.5881, -4.0864) centre (6.6825, -0.9126) ccw
  arc A23 (5.8245, -4.0008) -> (6.6045, -4.1168) centre (6.6825, -0.9126) ccw
  arc A24 (5.6703, -4.2165) -> (5.8245, -4.0008) centre (0, 0) ccw
  arc A25 (5.6334, -4.2158) -> (5.8119, -3.9661) centre (0, 0) ccw
  arc A26 (6.0325, -4.917) -> (5.6703, -4.2165) centre (3.0259, -6.0277) ccw
  arc A27 (5.9984, -4.9113) -> (5.6334, -4.2158) centre (3.0259, -6.0277) ccw
  arc A28 (3.0502, -6.3407) -> (3.6623, -6.8329) centre (5.3309, -4.1316) ccw
  arc A29 (2.7708, -6.4677) -> (3.0502, -6.3407) centre (0, 0) ccw
  arc A30 (2.7391, -7.2525) -> (2.7708, -6.4677) centre (-0.3933, -6.7331) ccw
  arc A31 (2.4201, -7.3651) -> (2.7391, -7.2525) centre (0, 0) ccw
  arc A32 (1.8902, -6.8087) -> (2.4131, -7.3989) centre (4.5325, -4.9945) ccw
  arc A33 (1.9029, -6.774) -> (2.4201, -7.3651) centre (4.5325, -4.9945) ccw
  arc A34 (2.4131, -7.3989) -> (2.7658, -7.2745) centre (0, 0) ccw
  arc A35 (2.7658, -7.2745) -> (2.8024, -6.4867) centre (-0.3933, -6.7331) ccw
  arc A36 (2.8024, -6.4867) -> (3.0438, -6.377) centre (0, 0) ccw
  arc A37 (3.0438, -6.377) -> (3.6613, -6.8675) centre (5.3309, -4.1316) ccw
  arc A38 (6.3164, -3.1678) -> (6.4308, -2.9286) centre (0, 0) ccw
  arc A39 (6.2799, -3.1735) -> (6.4123, -2.8966) centre (0, 0) ccw
  arc A40 (6.4308, -2.9286) -> (7.219, -2.9074) centre (6.7395, 0.2617) ccw
  arc A41 (6.4123, -2.8966) -> (7.1976, -2.8803) centre (6.7395, 0.2617) ccw
  arc A42 (7.219, -2.9074) -> (7.3504, -2.5572) centre (0, 0) ccw
  arc A43 (7.3164, -2.5636) -> (6.7356, -2.0348) centre (4.905, -4.6292) ccw
  arc A44 (7.3504, -2.5572) -> (6.7705, -2.0228) centre (4.905, -4.6292) ccw
  arc A45 (7.1976, -2.8803) -> (7.3164, -2.5636) centre (0, 0) ccw
  arc A46 (1.1044, -7.6734) -> (1.4381, -7.618) centre (0, 0) ccw
  arc A47 (0.6976, -7.0015) -> (1.1044, -7.6734) centre (3.5964, -5.7057) ccw
  arc A48 (-0.5525, -7.0446) -> (-0.263, -7.7781) centre (2.5509, -6.2435) ccw
  arc A49 (-0.5288, -7.0163) -> (-0.2448, -7.7487) centre (2.5509, -6.2435) ccw
  arc A50 (-0.2448, -7.7487) -> (0.0934, -7.752) centre (0, 0) ccw
  arc A51 (0.0934, -7.752) -> (0.3916, -7.0253) centre (-2.6724, -6.1925) ccw
  arc A52 (0.111, -7.7817) -> (0.4148, -7.054) centre (-2.6724, -6.1925) ccw
  arc A53 (0.4148, -7.054) -> (0.6792, -7.0335) centre (0, 0) ccw
  arc A54 (0.3916, -7.0253) -> (0.6976, -7.0015) centre (0, 0) ccw
  arc A55 (0.6792, -7.0335) -> (1.0916, -7.7056) centre (3.5964, -5.7057) ccw
  arc A56 (1.6056, -6.8506) -> (1.9029, -6.774) centre (0, 0) ccw
  arc A57 (1.6334, -6.8748) -> (1.8902, -6.8087) centre (0, 0) ccw
  arc A58 (1.4381, -7.618) -> (1.6056, -6.8506) centre (-1.5565, -6.5625) ccw
  arc A59 (1.4606, -7.6442) -> (1.6334, -6.8748) centre (-1.5565, -6.5625) ccw
  arc A60 (1.0916, -7.7056) -> (1.4606, -7.6442) centre (0, 0) ccw
  arc A61 (-0.263, -7.7781) -> (0.111, -7.7817) centre (0, 0) ccw
  arc A62 (-0.8164, -7.0189) -> (-0.5525, -7.0446) centre (0, 0) ccw
  arc A63 (-0.8343, -6.9866) -> (-0.5288, -7.0163) centre (0, 0) ccw
  arc A64 (-1.242, -7.6828) -> (-0.8164, -7.0189) centre (-3.7071, -5.6343) ccw
  arc A65 (-1.2541, -7.6504) -> (-0.8343, -6.9866) centre (-3.7071, -5.6343) ccw
  arc A66 (7.0253, 0.3916) -> (7.0015, 0.6976) centre (0, 0) ccw
  arc A67 (7.752, 0.0934) -> (7.0253, 0.3916) centre (6.1925, -2.6724) ccw
  arc A68 (7.7487, -0.2448) -> (7.752, 0.0934) centre (0, 0) ccw
  arc A69 (7.0163, -0.5288) -> (7.7487, -0.2448) centre (6.2435, 2.5509) ccw
  arc A70 (6.9866, -0.8343) -> (7.0163, -0.5288) centre (0, 0) ccw
  arc A71 (7.6504, -1.2541) -> (6.9866, -0.8343) centre (5.6343, -3.7071) ccw
  arc A72 (7.5884, -1.5866) -> (7.6504, -1.2541) centre (0, 0) ccw
  arc A73 (6.8179, -1.7391) -> (7.5884, -1.5866) centre (6.5916, 1.428) ccw
  arc A74 (6.7356, -2.0348) -> (6.8179, -1.7391) centre (0, 0) ccw
  arc A75 (6.8416, -1.7674) -> (7.6142, -1.6097) centre (6.5916, 1.428) ccw
  arc A76 (7.6142, -1.6097) -> (7.6828, -1.242) centre (0, 0) ccw
  arc A77 (7.0189, -0.8164) -> (7.0446, -0.5525) centre (0, 0) ccw
  arc A78 (7.6828, -1.242) -> (7.0189, -0.8164) centre (5.6343, -3.7071) ccw
  arc A79 (7.0446, -0.5525) -> (7.7781, -0.263) centre (6.2435, 2.5509) ccw
  arc A80 (7.7781, -0.263) -> (7.7817, 0.111) centre (0, 0) ccw
  arc A81 (7.7817, 0.111) -> (7.054, 0.4148) centre (6.1925, -2.6724) ccw
  arc A82 (7.054, 0.4148) -> (7.0335, 0.6792) centre (0, 0) ccw
  arc A83 (6.7705, -2.0228) -> (6.8416, -1.7674) centre (0, 0) ccw
  arc A84 (-2.8966, -6.4123) -> (-2.8803, -7.1976) centre (0.2617, -6.7395) ccw
  arc A85 (-2.8803, -7.1976) -> (-2.5636, -7.3164) centre (0, 0) ccw
  arc A86 (-2.9074, -7.219) -> (-2.5572, -7.3504) centre (0, 0) ccw
  arc A87 (-2.0228, -6.7705) -> (-1.7674, -6.8416) centre (0, 0) ccw
  arc A88 (-2.5636, -7.3164) -> (-2.0348, -6.7356) centre (-4.6292, -4.905) ccw
  arc A89 (-2.0348, -6.7356) -> (-1.7391, -6.8179) centre (0, 0) ccw
  arc A90 (-2.5572, -7.3504) -> (-2.0228, -6.7705) centre (-4.6292, -4.905) ccw
  arc A91 (-1.7391, -6.8179) -> (-1.5866, -7.5884) centre (1.428, -6.5916) ccw
  arc A92 (-1.7674, -6.8416) -> (-1.6097, -7.6142) centre (1.428, -6.5916) ccw
  arc A93 (-1.5866, -7.5884) -> (-1.2541, -7.6504) centre (0, 0) ccw
  arc A94 (-1.6097, -7.6142) -> (-1.242, -7.6828) centre (0, 0) ccw
  arc A95 (-2.9286, -6.4308) -> (-2.9074, -7.219) centre (0.2617, -6.7395) ccw
  arc A96 (-3.1678, -6.3164) -> (-2.9286, -6.4308) centre (0, 0) ccw
  arc A97 (-3.7947, -6.7947) -> (-3.1678, -6.3164) centre (-5.4106, -4.0266) ccw
  arc A98 (-3.7951, -6.7601) -> (-3.1735, -6.2799) centre (-5.4106, -4.0266) ccw
  arc A99 (-4.0864, -6.5881) -> (-3.7951, -6.7601) centre (0, 0) ccw
  arc A100 (-4.1168, -6.6045) -> (-3.7947, -6.7947) centre (0, 0) ccw
  arc A101 (-3.9661, -5.8119) -> (-4.0864, -6.5881) centre (-0.9126, -6.6825) ccw
  arc A102 (-4.0008, -5.8245) -> (-4.1168, -6.6045) centre (-0.9126, -6.6825) ccw
  arc A103 (-3.1735, -6.2799) -> (-2.8966, -6.4123) centre (0, 0) ccw
  arc A104 (6.4677, 2.7708) -> (6.3407, 3.0502) centre (0, 0) ccw
  arc A105 (7.2525, 2.7391) -> (6.4677, 2.7708) centre (6.7331, -0.3933) ccw
  arc A106 (7.3651, 2.4201) -> (7.2525, 2.7391) centre (0, 0) ccw
  arc A107 (6.774, 1.9029) -> (7.3651, 2.4201) centre (4.9945, 4.5325) ccw
  arc A108 (6.8506, 1.6056) -> (6.774, 1.9029) centre (0, 0) ccw
  arc A109 (7.618, 1.4381) -> (6.8506, 1.6056) centre (6.5625, -1.5565) ccw
  arc A110 (7.6734, 1.1044) -> (7.618, 1.4381) centre (0, 0) ccw
  arc A111 (7.0015, 0.6976) -> (7.6734, 1.1044) centre (5.7057, 3.5964) ccw
  arc A112 (6.4867, 2.8024) -> (6.377, 3.0438) centre (0, 0) ccw
  arc A113 (6.8748, 1.6334) -> (6.8087, 1.8902) centre (0, 0) ccw
  arc A114 (7.2745, 2.7658) -> (6.4867, 2.8024) centre (6.7331, -0.3933) ccw
  arc A115 (7.3989, 2.4131) -> (7.2745, 2.7658) centre (0, 0) ccw
  arc A116 (6.8087, 1.8902) -> (7.3989, 2.4131) centre (4.9945, 4.5325) ccw
  arc A117 (7.6442, 1.4606) -> (6.8748, 1.6334) centre (6.5625, -1.5565) ccw
  arc A118 (7.0335, 0.6792) -> (7.7056, 1.0916) centre (5.7057, 3.5964) ccw
  arc A119 (7.7056, 1.0916) -> (7.6442, 1.4606) centre (0, 0) ccw
  arc A120 (-4.2158, -5.6334) -> (-3.9661, -5.8119) centre (0, 0) ccw
  arc A121 (-4.9113, -5.9984) -> (-4.2158, -5.6334) centre (-6.0277, -3.0259) ccw
  arc A122 (-5.1683, -5.7784) -> (-4.9113, -5.9984) centre (0, 0) ccw
  arc A123 (-4.915, -5.0349) -> (-5.1683, -5.7784) centre (-2.0591, -6.4225) ccw
  arc A124 (-5.13, -4.8157) -> (-4.915, -5.0349) centre (0, 0) ccw
  arc A125 (-5.8783, -5.0544) -> (-5.13, -4.8157) centre (-6.4615, -1.9333) ccw
  arc A126 (-6.0932, -4.7932) -> (-5.8783, -5.0544) centre (0, 0) ccw
  arc A127 (-5.7147, -4.1049) -> (-6.0932, -4.7932) centre (-3.1431, -5.9674) ccw
  arc A128 (-5.8883, -3.8518) -> (-5.7147, -4.1049) centre (0, 0) ccw
  arc A129 (-5.9016, -3.8862) -> (-5.7516, -4.1049) centre (0, 0) ccw
  arc A130 (-5.7516, -4.1049) -> (-6.1274, -4.7982) centre (-3.1431, -5.9674) ccw
  arc A131 (-6.1274, -4.7982) -> (-5.8898, -5.087) centre (0, 0) ccw
  arc A132 (-5.8898, -5.087) -> (-5.1371, -4.852) centre (-6.4615, -1.9333) ccw
  arc A133 (-5.1371, -4.852) -> (-4.9514, -5.0413) centre (0, 0) ccw
  arc A134 (-4.9514, -5.0413) -> (-5.2011, -5.7893) centre (-2.0591, -6.4225) ccw
  arc A135 (-5.2011, -5.7893) -> (-4.917, -6.0325) centre (0, 0) ccw
  arc A136 (-4.2165, -5.6703) -> (-4.0008, -5.8245) centre (0, 0) ccw
  arc A137 (-4.917, -6.0325) -> (-4.2165, -5.6703) centre (-6.0277, -3.0259) ccw
  arc A138 (4.915, 5.0349) -> (5.1683, 5.7784) centre (2.0591, 6.4225) ccw
  arc A139 (5.13, 4.8157) -> (4.915, 5.0349) centre (0, 0) ccw
  arc A140 (5.8783, 5.0544) -> (5.13, 4.8157) centre (6.4615, 1.9333) ccw
  arc A141 (6.0932, 4.7932) -> (5.8783, 5.0544) centre (0, 0) ccw
  arc A142 (5.7147, 4.1049) -> (6.0932, 4.7932) centre (3.1431, 5.9674) ccw
  arc A143 (5.8883, 3.8518) -> (5.7147, 4.1049) centre (0, 0) ccw
  arc A144 (6.6667, 3.9569) -> (5.8883, 3.8518) centre (6.6991, 0.7819) ccw
  arc A145 (6.8329, 3.6623) -> (6.6667, 3.9569) centre (0, 0) ccw
  arc A146 (6.3407, 3.0502) -> (6.8329, 3.6623) centre (4.1316, 5.3309) ccw
  arc A147 (6.377, 3.0438) -> (6.8675, 3.6613) centre (4.1316, 5.3309) ccw
  arc A148 (6.8675, 3.6613) -> (6.6837, 3.987) centre (0, 0) ccw
  arc A149 (6.6837, 3.987) -> (5.9016, 3.8862) centre (6.6991, 0.7819) ccw
  arc A150 (5.9016, 3.8862) -> (5.7516, 4.1049) centre (0, 0) ccw
  arc A151 (6.1274, 4.7982) -> (5.8898, 5.087) centre (0, 0) ccw
  arc A152 (5.8898, 5.087) -> (5.1371, 4.852) centre (6.4615, 1.9333) ccw
  arc A153 (5.1371, 4.852) -> (4.9514, 5.0413) centre (0, 0) ccw
  arc A154 (4.9514, 5.0413) -> (5.2011, 5.7893) centre (2.0591, 6.4225) ccw
  arc A155 (5.7516, 4.1049) -> (6.1274, 4.7982) centre (3.1431, 5.9674) ccw
  arc A156 (-6.6667, -3.9569) -> (-5.8883, -3.8518) centre (-6.6991, -0.7819) ccw
  arc A157 (-6.8329, -3.6623) -> (-6.6667, -3.9569) centre (0, 0) ccw
  arc A158 (-6.3407, -3.0502) -> (-6.8329, -3.6623) centre (-4.1316, -5.3309) ccw
  arc A159 (-6.4677, -2.7708) -> (-6.3407, -3.0502) centre (0, 0) ccw
  arc A160 (-7.2525, -2.7391) -> (-6.4677, -2.7708) centre (-6.7331, 0.3933) ccw
  arc A161 (-7.3651, -2.4201) -> (-7.2525, -2.7391) centre (0, 0) ccw
  arc A162 (-6.774, -1.9029) -> (-7.3651, -2.4201) centre (-4.9945, -4.5325) ccw
  arc A163 (-6.8506, -1.6056) -> (-6.774, -1.9029) centre (0, 0) ccw
  arc A164 (-6.8748, -1.6334) -> (-6.8087, -1.8902) centre (0, 0) ccw
  arc A165 (-6.8087, -1.8902) -> (-7.3989, -2.4131) centre (-4.9945, -4.5325) ccw
  arc A166 (-7.3989, -2.4131) -> (-7.2745, -2.7658) centre (0, 0) ccw
  arc A167 (-7.2745, -2.7658) -> (-6.4867, -2.8024) centre (-6.7331, 0.3933) ccw
  arc A168 (-6.4867, -2.8024) -> (-6.377, -3.0438) centre (0, 0) ccw
  arc A169 (-6.377, -3.0438) -> (-6.8675, -3.6613) centre (-4.1316, -5.3309) ccw
  arc A170 (-6.6837, -3.987) -> (-5.9016, -3.8862) centre (-6.6991, -0.7819) ccw
  arc A171 (-6.8675, -3.6613) -> (-6.6837, -3.987) centre (0, 0) ccw
  arc A172 (2.8803, 7.1976) -> (2.5636, 7.3164) centre (0, 0) ccw
  arc A173 (2.8966, 6.4123) -> (2.8803, 7.1976) centre (-0.2617, 6.7395) ccw
  arc A174 (3.1735, 6.2799) -> (2.8966, 6.4123) centre (0, 0) ccw
  arc A175 (3.7951, 6.7601) -> (3.1735, 6.2799) centre (5.4106, 4.0266) ccw
  arc A176 (4.0864, 6.5881) -> (3.7951, 6.7601) centre (0, 0) ccw
  arc A177 (3.9661, 5.8119) -> (4.0864, 6.5881) centre (0.9126, 6.6825) ccw
  arc A178 (4.2158, 5.6334) -> (3.9661, 5.8119) centre (0, 0) ccw
  arc A179 (4.9113, 5.9984) -> (4.2158, 5.6334) centre (6.0277, 3.0259) ccw
  arc A180 (5.1683, 5.7784) -> (4.9113, 5.9984) centre (0, 0) ccw
  arc A181 (5.2011, 5.7893) -> (4.917, 6.0325) centre (0, 0) ccw
  arc A182 (4.917, 6.0325) -> (4.2165, 5.6703) centre (6.0277, 3.0259) ccw
  arc A183 (4.2165, 5.6703) -> (4.0008, 5.8245) centre (0, 0) ccw
  arc A184 (4.0008, 5.8245) -> (4.1168, 6.6045) centre (0.9126, 6.6825) ccw
  arc A185 (4.1168, 6.6045) -> (3.7947, 6.7947) centre (0, 0) ccw
  arc A186 (3.1678, 6.3164) -> (2.9286, 6.4308) centre (0, 0) ccw
  arc A187 (3.7947, 6.7947) -> (3.1678, 6.3164) centre (5.4106, 4.0266) ccw
  arc A188 (2.9286, 6.4308) -> (2.9074, 7.219) centre (-0.2617, 6.7395) ccw
  arc A189 (2.9074, 7.219) -> (2.5572, 7.3504) centre (0, 0) ccw
  arc A190 (0.2448, 7.7487) -> (-0.0934, 7.752) centre (0, 0) ccw
  arc A191 (0.5288, 7.0163) -> (0.2448, 7.7487) centre (-2.5509, 6.2435) ccw
  arc A192 (0.8343, 6.9866) -> (0.5288, 7.0163) centre (0, 0) ccw
  arc A193 (1.2541, 7.6504) -> (0.8343, 6.9866) centre (3.7071, 5.6343) ccw
  arc A194 (1.5866, 7.5884) -> (1.2541, 7.6504) centre (0, 0) ccw
  arc A195 (1.7391, 6.8179) -> (1.5866, 7.5884) centre (-1.428, 6.5916) ccw
  arc A196 (2.0348, 6.7356) -> (1.7391, 6.8179) centre (0, 0) ccw
  arc A197 (2.5636, 7.3164) -> (2.0348, 6.7356) centre (4.6292, 4.905) ccw
  arc A198 (2.5572, 7.3504) -> (2.0228, 6.7705) centre (4.6292, 4.905) ccw
  arc A199 (2.0228, 6.7705) -> (1.7674, 6.8416) centre (0, 0) ccw
  arc A200 (1.6097, 7.6142) -> (1.242, 7.6828) centre (0, 0) ccw
  arc A201 (0.8164, 7.0189) -> (0.5525, 7.0446) centre (0, 0) ccw
  arc A202 (1.242, 7.6828) -> (0.8164, 7.0189) centre (3.7071, 5.6343) ccw
  arc A203 (0.5525, 7.0446) -> (0.263, 7.7781) centre (-2.5509, 6.2435) ccw
  arc A204 (0.263, 7.7781) -> (-0.111, 7.7817) centre (0, 0) ccw
  arc A205 (1.7674, 6.8416) -> (1.6097, 7.6142) centre (-1.428, 6.5916) ccw
  circle A206 centre (0, 0) radius 8.5 construction
  arc A207 (-2.7391, 7.2525) -> (-2.7708, 6.4677) centre (0.3933, 6.7331) ccw
  arc A208 (-2.4201, 7.3651) -> (-2.7391, 7.2525) centre (0, 0) ccw
  arc A209 (-1.9029, 6.774) -> (-2.4201, 7.3651) centre (-4.5325, 4.9945) ccw
  arc A210 (-1.6056, 6.8506) -> (-1.9029, 6.774) centre (0, 0) ccw
  arc A211 (-1.4381, 7.618) -> (-1.6056, 6.8506) centre (1.5565, 6.5625) ccw
  arc A212 (-1.1044, 7.6734) -> (-1.4381, 7.618) centre (0, 0) ccw
  arc A213 (-0.6976, 7.0015) -> (-1.1044, 7.6734) centre (-3.5964, 5.7057) ccw
  arc A214 (-0.3916, 7.0253) -> (-0.6976, 7.0015) centre (0, 0) ccw
  arc A215 (-0.0934, 7.752) -> (-0.3916, 7.0253) centre (2.6724, 6.1925) ccw
  arc A216 (-0.111, 7.7817) -> (-0.4148, 7.054) centre (2.6724, 6.1925) ccw
  arc A217 (-0.4148, 7.054) -> (-0.6792, 7.0335) centre (0, 0) ccw
  arc A218 (-0.6792, 7.0335) -> (-1.0916, 7.7056) centre (-3.5964, 5.7057) ccw
  arc A219 (-1.0916, 7.7056) -> (-1.4606, 7.6442) centre (0, 0) ccw
  arc A220 (-1.4606, 7.6442) -> (-1.6334, 6.8748) centre (1.5565, 6.5625) ccw
  arc A221 (-1.6334, 6.8748) -> (-1.8902, 6.8087) centre (0, 0) ccw
  arc A222 (-1.8902, 6.8087) -> (-2.4131, 7.3989) centre (-4.5325, 4.9945) ccw
  arc A223 (-2.4131, 7.3989) -> (-2.7658, 7.2745) centre (0, 0) ccw
  arc A224 (-2.7658, 7.2745) -> (-2.8024, 6.4867) centre (0.3933, 6.7331) ccw
  arc A225 (-7.618, -1.4381) -> (-6.8506, -1.6056) centre (-6.5625, 1.5565) ccw
  arc A226 (-7.6734, -1.1044) -> (-7.618, -1.4381) centre (0, 0) ccw
  arc A227 (-7.0015, -0.6976) -> (-7.6734, -1.1044) centre (-5.7057, -3.5964) ccw
  arc A228 (-7.0253, -0.3916) -> (-7.0015, -0.6976) centre (0, 0) ccw
  arc A229 (-7.752, -0.0934) -> (-7.0253, -0.3916) centre (-6.1925, 2.6724) ccw
  arc A230 (-7.7487, 0.2448) -> (-7.752, -0.0934) centre (0, 0) ccw
  arc A231 (-7.0163, 0.5288) -> (-7.7487, 0.2448) centre (-6.2435, -2.5509) ccw
  arc A232 (-6.9866, 0.8343) -> (-7.0163, 0.5288) centre (0, 0) ccw
  arc A233 (-7.0189, 0.8164) -> (-7.0446, 0.5525) centre (0, 0) ccw
  arc A234 (-7.0446, 0.5525) -> (-7.7781, 0.263) centre (-6.2435, -2.5509) ccw
  arc A235 (-7.7781, 0.263) -> (-7.7817, -0.111) centre (0, 0) ccw
  arc A236 (-7.7817, -0.111) -> (-7.054, -0.4148) centre (-6.1925, 2.6724) ccw
  arc A237 (-7.054, -0.4148) -> (-7.0335, -0.6792) centre (0, 0) ccw
  arc A238 (-7.0335, -0.6792) -> (-7.7056, -1.0916) centre (-5.7057, -3.5964) ccw
  arc A239 (-7.7056, -1.0916) -> (-7.6442, -1.4606) centre (0, 0) ccw
  arc A240 (-7.6442, -1.4606) -> (-6.8748, -1.6334) centre (-6.5625, 1.5565) ccw
  arc A241 (-5.0544, 5.8783) -> (-4.8157, 5.13) centre (-1.9333, 6.4615) ccw
  arc A242 (-4.7932, 6.0932) -> (-5.0544, 5.8783) centre (0, 0) ccw
  arc A243 (-4.1049, 5.7147) -> (-4.7932, 6.0932) centre (-5.9674, 3.1431) ccw
  arc A244 (-3.8518, 5.8883) -> (-4.1049, 5.7147) centre (0, 0) ccw
  arc A245 (-3.9569, 6.6667) -> (-3.8518, 5.8883) centre (-0.7819, 6.6991) ccw
  arc A246 (-3.6623, 6.8329) -> (-3.9569, 6.6667) centre (0, 0) ccw
  arc A247 (-3.0502, 6.3407) -> (-3.6623, 6.8329) centre (-5.3309, 4.1316) ccw
  arc A248 (-2.7708, 6.4677) -> (-3.0502, 6.3407) centre (0, 0) ccw
  arc A249 (-2.8024, 6.4867) -> (-3.0438, 6.377) centre (0, 0) ccw
  arc A250 (-3.0438, 6.377) -> (-3.6613, 6.8675) centre (-5.3309, 4.1316) ccw
  arc A251 (-3.6613, 6.8675) -> (-3.987, 6.6837) centre (0, 0) ccw
  arc A252 (-3.987, 6.6837) -> (-3.8862, 5.9016) centre (-0.7819, 6.6991) ccw
  arc A253 (-3.8862, 5.9016) -> (-4.1049, 5.7516) centre (0, 0) ccw
  arc A254 (-4.1049, 5.7516) -> (-4.7982, 6.1274) centre (-5.9674, 3.1431) ccw
  arc A255 (-4.7982, 6.1274) -> (-5.087, 5.8898) centre (0, 0) ccw
  arc A256 (-5.087, 5.8898) -> (-4.852, 5.1371) centre (-1.9333, 6.4615) ccw
  arc A257 (-6.7601, 3.7951) -> (-6.2799, 3.1735) centre (-4.0266, 5.4106) ccw
  arc A258 (-6.5881, 4.0864) -> (-6.7601, 3.7951) centre (0, 0) ccw
  arc A259 (-5.8119, 3.9661) -> (-6.5881, 4.0864) centre (-6.6825, 0.9126) ccw
  arc A260 (-5.6334, 4.2158) -> (-5.8119, 3.9661) centre (0, 0) ccw
  arc A261 (-5.9984, 4.9113) -> (-5.6334, 4.2158) centre (-3.0259, 6.0277) ccw
  arc A262 (-5.7784, 5.1683) -> (-5.9984, 4.9113) centre (0, 0) ccw
  arc A263 (-5.0349, 4.915) -> (-5.7784, 5.1683) centre (-6.4225, 2.0591) ccw
  arc A264 (-4.8157, 5.13) -> (-5.0349, 4.915) centre (0, 0) ccw
  arc A265 (-4.852, 5.1371) -> (-5.0413, 4.9514) centre (0, 0) ccw
  arc A266 (-5.0413, 4.9514) -> (-5.7893, 5.2011) centre (-6.4225, 2.0591) ccw
  arc A267 (-5.7893, 5.2011) -> (-6.0325, 4.917) centre (0, 0) ccw
  arc A268 (-5.6703, 4.2165) -> (-5.8245, 4.0008) centre (0, 0) ccw
  arc A269 (-5.8245, 4.0008) -> (-6.6045, 4.1168) centre (-6.6825, 0.9126) ccw
  arc A270 (-6.6045, 4.1168) -> (-6.7947, 3.7947) centre (0, 0) ccw
  arc A271 (-6.7947, 3.7947) -> (-6.3164, 3.1678) centre (-4.0266, 5.4106) ccw
  arc A272 (-6.0325, 4.917) -> (-5.6703, 4.2165) centre (-3.0259, 6.0277) ccw
  arc A273 (-7.6504, 1.2541) -> (-6.9866, 0.8343) centre (-5.6343, 3.7071) ccw
  arc A274 (-7.5884, 1.5866) -> (-7.6504, 1.2541) centre (0, 0) ccw